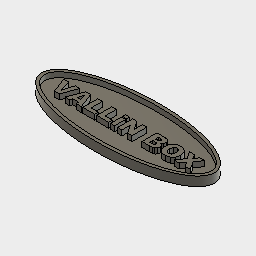
Logo Vallin Box (Autodesk Fusion 360 design; units mm, degrees)
Autodesk Fusion 360 part; units mm, degrees
note: some values were not read from the file. Chosen so that the rebuilt part matches the saved one: which bodies a step acts on.
sketch "Sketch1" plane through (0, 0, 0) normal (0, 1, 0) x (1, 0, 0)
  ellipse E0 centre (0, 0) end of major axis (66.5407, 0) minor radius 24.757
  line L0 (-66.5407, 0) -> (66.5407, 0)
  line L1 (0, -24.757) -> (0, 24.757)
  ellipse E1 centre (0, 0) end of major axis (64.1367, 0) minor radius 22.353
  line L2 (-53.7463, -7.3372) -> (55.0308, -7.3372) construction
  line L3 (55.0308, -7.3372) -> (55.0308, 8.7129) construction
  line L4 (55.0308, 8.7129) -> (-53.7463, 8.7129) construction
  line L5 (-53.7463, 8.7129) -> (-53.7463, -7.3372) construction
  text T0 "VALLiN BOX" font "Arial Black" height 16.0501 align ink ink in box 0 x 0 at (-53.7363, -7.3172) x (1, 0) y (0, 1) spacing 1 height is em
extrude "Extrude1" add sketch "Sketch1" sketch "Sketch1" along normal blind 4 contours E0 L0 L1 E1 | E0 L0 L1 E1 | E0 L0 L1 E1 | E0 L0 L1 E1 of sketch 2 text T0 makes body 1 at (-31.8816, 0, 1.8314) makes body 2 at (-15.7427, 0, 2.3486) makes body 3 at (-5.2516, 1.3333, -4.3677) makes body 4 at (19.0482, 0, 1.6929) makes body 5 at (-4.3388, 2.6667, 24.7044) makes body 6 at (52.4076, 0, 5.1464) makes body 7 at (-3.1252, 1.3333, 1.5728) makes body 8 at (31.1202, 0, 0.7032) makes body 9 at (-26.448, 0, 2.3486) makes body 10 at (-50.1888, 0, 2.218) makes body 11 at (9.0195, 0, 1.5806)
extrude "Extrude2" add sketch "Sketch1" against normal blind 4 separate body makes body 12
extrude "Extrude3" cut 1 faces at (-0.892, -4, 8.0909) along direction (0, 1, 0) blind 1 on bodies 12 bodies 12
combine "Combine1" operation add target body 1 tool bodies 11 3 9 6 5 7 4 12 2 8 10
